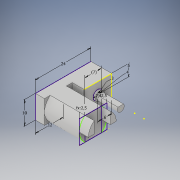
# Autodesk Inventor part: motorcek
Saved by Autodesk Inventor 2019 (Build 230136000, 136)
## iProperties
Created: 2020-07-24
Part Number: motorcek
Material: Generic
Document SubType Name: Modeling
Designer: lukad
Density: 1 g/cm^3
Appearance: Default
Author: lukad
Autodesk Inventor part; units mm, degrees
ref_plane "YZ Plane" through (0, 0, 0) normal (1, 0, 0) x (0, 1, 0)
ref_plane "XZ Plane" through (0, 0, 0) normal (0, 1, 0) x (-1, 0, 0)
ref_plane "XY Plane" through (0, 0, 0) normal (0, 0, 1) x (1, 0, 0)
sketch "Sketch1" plane through (0, 0, 0) normal (1, 0, 0) x (0, 1, 0)
  line L0 (10, 24) -> (0, 24)
  line L1 (0, 24) -> (0, 0)
  line L2 (0, 0) -> (10, 0)
  line L3 (10, 0) -> (10, 24)
  line L4 (10, 24) -> (0, 24)
  line L5 (0, 24) -> (0, 12)
  line L6 (0, 12) -> (10, 12)
  line L7 (10, 12) -> (10, 24)
  dimension "d0" = 24
  dimension "d1" = 10
  dimension "d2" = 12
  constraints: 16 end point, 4 parallel, 2 horizontal, 2 perpendicular, 1 midpoint
  measures "d0" distance of L2.end L0.start
  measures "d1" distance of L0.start L0.end
  measures "d2" distance between parallel lines of L6 L0
extrude "Extrusion1" add sketch "Sketch1" along normal blind 19 contours L3 L6 L1 L0
extrude "Extrusion2" add sketch "Sketch1" along normal blind 9 contours L3 L2 L1 L6
sketch "Sketch2" plane through (9, 0, 0) normal (1, 0, 0) x (0, 0, -1)
  circle A0 centre (-6, 5) radius 2
  line L0 (0, 10) -> (-12, 10) projected
  line L1 (0, 0) -> (0, 10) projected
  circle A1 centre (-6, 5) radius 1.5
  line L2 (-7.2, 5.9) -> (-4.8, 5.9)
  dimension "d7" = 4
  dimension "d8" = 5
  dimension "d9" = 6
  dimension "d10" = 3
  dimension "d11" = 2.4
  constraints: 2 centre point, 2 end point, 2 point on circle, 1 concentric, 1 horizontal
  measures "d7" diameter of A0
  measures "d8" distance from line of L0 A0.centre
  measures "d9" distance from line of L1 A0.centre
  measures "d10" diameter of A1
extrude "Extrusion3" add sketch "Sketch2" along normal blind 1
extrude "Extrusion4" add sketch "Sketch2" along normal blind 10 contours A1 L2 picked at (-5.5775, 4.8311)
extrude "Extrusion5" add sketch "Sketch2" along normal blind 1 contours L2 A1 picked at (-5.6796, 5.9839)
sketch "Sketch3" plane through (19, 0, 0) normal (1, 0, 0) x (0, 0, -1)
  line L0 (-24, 10) -> (-24, 0) projected
  line L1 (-24, 10) -> (-12, 10)
  line L2 (-12, 10) -> (-12, 0)
  line L3 (-12, 0) -> (-24, 0)
  line L4 (-24, 0) -> (-24, 10)
  line L5 (-12, 10) -> (-24, 10) projected
  line L6 (-24, 0) -> (-12, 0) projected
  line L7 (-21.5, 10) -> (-14.5, 10)
  line L8 (-14.5, 10) -> (-14.5, 0)
  line L9 (-14.5, 0) -> (-21.5, 0)
  line L10 (-21.5, 0) -> (-21.5, 10)
  arc A0 (-21.5, 10) -> (-21.5, 0) centre (-17.75, 5) ccw
  arc A1 (-14.5, 0) -> (-14.5, 10) centre (-18.25, 5) ccw
  point P0 (0, 0)
  dimension "d18" = 2.5
  dimension "d19" = 2.5
  dimension "d20" = 7
  constraints: 16 end point, 4 parallel, 4 point on circle, 2 centre point, 2 horizontal, 2 perpendicular, 2 point on line
  measures "d18" distance between parallel lines of L2 L8
  measures "d19" distance between parallel lines of L0 L10
  measures "d20" distance between parallel lines of L8 L10
extrude "Extrusion6" cut sketch "Sketch3" against normal blind 15 contours L1 A0 L0 | A0 L3 L0
extrude "Extrusion7" cut sketch "Sketch3" against normal blind 15 contours L1 L2 A1 | A1 L2 L3
extrude "Extrusion8" add sketch "Sketch3" along normal blind 4 contours A0 L10 | L1 L8 L3 L10 | A1 L8
sketch "Sketch4" plane through (23, 0, 0) normal (1, 0, 0) x (0, 0, -1)
  line L0 (-12, 5) -> (-12, 0) projected
  line L1 (-23.9948, 0) -> (-12, 0)
  line L2 (-12, 0) -> (-12, 5)
  line L3 (-12, 5) -> (-23.9948, 5)
  line L4 (-23.9948, 5) -> (-23.9948, 0)
  point P0 (0, 0)
  constraints: 8 end point, 2 parallel, 1 horizontal, 1 perpendicular
extrude "Extrusion9" cut sketch "Sketch4" against normal blind 4
sketch "Sketch5" plane through (23, 0, 0) normal (1, 0, 0) x (0, 0, -1)
  point P0 (0, 0)
sketch "Sketch6" plane through (0, 10, 0) normal (0, 1, 0) x (1, 0, 0)
  line L0 (23, -23.9948) -> (23, -12) projected
  line L1 (19, -12) -> (19, -14.5) projected
  line L2 (23, -21.4808) -> (19, -21.4808)
  line L3 (19, -21.4808) -> (19, -14.5)
  line L4 (19, -14.5) -> (23, -14.5)
  line L5 (23, -14.5) -> (23, -21.4808)
  point P0 (0, 0)
  constraints: 8 end point, 2 parallel, 1 horizontal, 1 perpendicular, 1 point on line
extrude "Extrusion10" cut sketch "Sketch6" against normal blind 8
equation "\"d19\" = d18"
body "Solid1"
